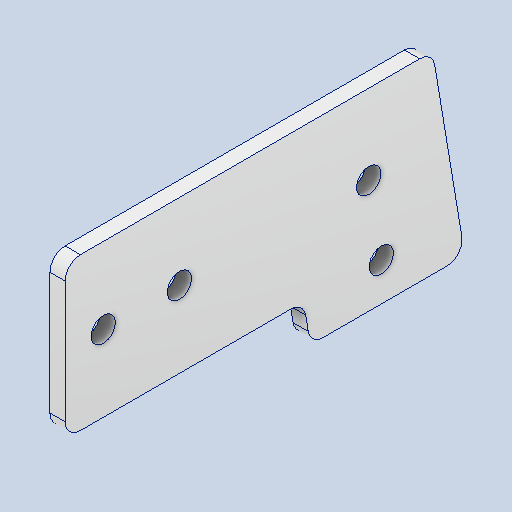
# Autodesk Inventor part: dribl-v3-Plate-12
Saved by Autodesk Inventor 2025.2 (Build 292293000, 293)
## iProperties
Created: 2025-04-05
Part Number: dribl-v3-Plate-12
Material: アルミニウム 6061
Document SubType Name: Modeling
Designer: haruy
Density: 2.7 g/cm^3
Appearance: アルミニウム - フラット
Author: haruy
Autodesk Inventor part; units mm, degrees
ref_plane "YZ Plane" through (0, 0, 0) normal (1, 0, 0) x (0, 1, 0)
ref_plane "XZ Plane" through (0, 0, 0) normal (0, 1, 0) x (-1, 0, 0)
ref_plane "XY Plane" through (0, 0, 0) normal (0, 0, 1) x (1, 0, 0)
derived "dribl-v3-Sketch-Base.ipt"
sketch "スケッチ9" plane through (400, -232.3334, -323) normal (1, 0, 0) x (0, 0, -1)
  line L0 (0, 20) -> (255, 20) projected
  line L1 (235, 20) -> (235, 0) projected
  line L2 (0, 0) -> (255, 0) projected
  line L3 (255, 0) -> (255, 20) projected
  line L4 (255, 20) -> (262.9654, 20) projected
  line L5 (64.2746, 1209.2041) -> (299.1068, -196.3132) projected
  line L6 (262.9654, 20) -> (282.2288, 20) projected
  line L7 (317.847, -193.1821) -> (83.0148, 1212.3352) projected
  line L8 (255, 0) -> (266.307, 0) projected
  circle A0 centre (240, 10) radius 1.6 projected
  circle A1 centre (250, 10) radius 1.6 projected
  circle A2 centre (274.8576, 9.5046) radius 1.6 projected
  line L9 (299.1068, -196.3132) -> (318.8333, -193.0173) projected
  circle A3 centre (276.5055, -0.3586) radius 1.6 projected
  line L10 (267.2023, -5.3586) -> (287.4795, -5.3586) projected
  line L11 (318.8333, -193.0173) -> (84.0011, 1212.5) projected
  line L12 (266.307, 0) -> (267.2023, -5.3586) projected
  line L13 (299.1068, -196.3132) -> (64.2746, 1209.2041) projected
  line L14 (282.2288, 20) -> (283.2427, 20) projected
  line L15 (283.2427, 20) -> (287.4795, -5.3586) projected
  point P0 (-323, 232.3334)
extrude "押し出し1" add sketch "スケッチ9" against normal blind 2 contours L0 L3 L2 L1 | L4 L5 L8 L3 | L6 L7 L10 L5 | L14 L11 L10 L7
fillet "フィレット1" radius 2 6 edges at (399, -212.3334, -558) (399, -232.3334, -558) (399, -232.3334, -589.307) (399, -237.692, -590.2023) (399, -237.692, -610.4795) (399, -212.3334, -606.2427)
